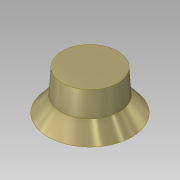
# Autodesk Inventor part: Knob
Saved by Autodesk Inventor 2016 (Build 200138000, 138)
## iProperties
Created: 2018-09-08
Part Number: Knob
Material: Generic
Document SubType Name: Modeling
Designer: Pedro Mendonça
Density: 1 g/cm^3
Appearance: Gold - Metal
Author: Pedro Mendonça
Autodesk Inventor part; units mm, degrees
ref_plane "XZ Plane" through (0, 0, 0) normal (0, 1, 0) x (-1, 0, 0)
ref_plane "XY Plane" through (0, 0, 0) normal (0, 0, 1) x (1, 0, 0)
sketch "Sketch1" plane through (0, 0, 0) normal (1, 0, 0) x (0, 1, 0)
  line L0 (0, 0) -> (0, 12.45)
  line L1 (0, 12.45) -> (8.7, 12.45)
  line L2 (8.7, 12.45) -> (9.2, 4.8665)
  line L3 (0, 0) -> (13.15, 0)
  line L4 (13.15, 0) -> (9.2, 4.8665)
  line L5 (0, -2.49) -> (0, 14.94) projected
  dimension "d5" = 12.45
  dimension "d6" = 8.7
  dimension "d7" = 7.6
  dimension "d8" = 13.15
  dimension "d10" = 9.2
  constraints: 10 end point, 1 horizontal, 1 perpendicular, 1 vertical
  measures "d5" distance of L0.start L0.end
  measures "d6" distance of L0.end L1.end
  measures "d7" distance of L1.end L2.end
  measures "d8" distance of L0.start L3.end
  measures "d10" distance from line of L2.end L0
revolve "Revolution1" add sketch "Sketch1" angle 360 about axis through (0, 0, -10) along (0, 0, 1)
sketch "Sketch2" plane through (0, 0, 0) normal (1, 0, 0) x (0, 1, 0)
  line L0 (-11.15, 0) -> (-7.2104, 4.8749)
  line L1 (-7.2173, 4.8665) -> (-6.8225, 10.8535)
  line L2 (-6.8225, 10.8535) -> (-4.8225, 10.8535)
  line L3 (-4.8225, 10.8535) -> (-4.8225, 0)
  line L4 (-11.15, 0) -> (-4.8225, 0)
  line L5 (-13.15, 0) -> (13.15, 0) projected
  line L6 (-11.15, 0) -> (-7.2173, 4.8665)
  line L7 (-6.8225, 10.8535) -> (-4.8225, 10.8535)
  line L8 (-4.8225, 0) -> (-11.15, 0)
  line L9 (0, -2.49) -> (0, 14.94) projected
  point P0 (0, 0)
  dimension "d14" = 6
  dimension "d15" = 2
  constraints: 16 end point, 2 horizontal, 2 parallel, 1 collinear
  measures "d14" distance of L1.start L1.end
  measures "d15" distance of L1.end L2.end
revolve "Revolution2" cut sketch "Sketch2" angle 360 about axis through (0, 0, -10) along (0, 0, 1)
sketch "Sketch3" plane through (0, 0, 0) normal (0, 0, -1) x (-1, 0, 0)
  circle A0 centre (0, 0) radius 3.125
  dimension "d17" = 6.25
  constraints: 1 centre point, 1 coincident
  measures "d17" diameter of A0
extrude "Extrusion1" cut sketch "Sketch3" against normal blind 8
sketch "Sketch4" plane through (0, 0, 0) normal (0, 0, -1) x (-1, 0, 0)
  circle A0 centre (0, 0) radius 3.125 projected
  circle A1 centre (0, -3.125) radius 0.485
  circle A2 centre (0.9657, -2.9721) radius 0.485
  circle A3 centre (1.8368, -2.5282) radius 0.485
  circle A4 centre (2.5282, -1.8368) radius 0.485
  circle A5 centre (2.9721, -0.9657) radius 0.485
  circle A6 centre (3.125, 0) radius 0.485
  circle A7 centre (2.9721, 0.9657) radius 0.485
  circle A8 centre (2.5282, 1.8368) radius 0.485
  circle A9 centre (1.8368, 2.5282) radius 0.485
  circle A10 centre (0.9657, 2.9721) radius 0.485
  circle A11 centre (0, 3.125) radius 0.485
  circle A12 centre (-0.9657, 2.9721) radius 0.485
  circle A13 centre (-1.8368, 2.5282) radius 0.485
  circle A14 centre (-2.5282, 1.8368) radius 0.485
  circle A15 centre (-2.9721, 0.9657) radius 0.485
  circle A16 centre (-3.125, 0) radius 0.485
  circle A17 centre (-2.9721, -0.9657) radius 0.485
  circle A18 centre (-2.5282, -1.8368) radius 0.485
  circle A19 centre (-1.8368, -2.5282) radius 0.485
  circle A20 centre (-0.9657, -2.9721) radius 0.485
  dimension "d20" = 0.97
  dimension "d23" = 360
  constraints: 20 centre point, 1 vertical alignment, 42 other
  measures "d20" diameter of A1
extrude "Extrusion2" cut sketch "Sketch4" against normal blind 8 contours A0 A6 | A0 A6 | A7 A0 | A0 A7 | A5 A0 | A0 A5 | A8 A0 | A0 A8 | A4 A0 | A0 A4 | A9 A0 | A0 A9 | A3 A0 | A0 A3 | A10 A0 | A0 A10 | A2 A0 | A0 A2 | A11 A0 | A0 A11 | A1 A0 | A0 A1 | A12 A0 | A0 A12 | A20 A0 | A0 A20 | A13 A0 | A0 A13 | A19 A0 | A0 A19 | A14 A0 | A0 A14 | A18 A0 | A0 A18 | A15 A0 | A0 A15 | A17 A0 | A0 A17 | A16 A0 | A0 A16
ref_plane "Work Plane1" through (15, 0, 0) normal (1, 0, 0) x (0, 1, 0)
sketch "Sketch5" plane through (15, 0, 0) normal (1, 0, 0) x (0, 1, 0)
  line L0 (-13.15, 0) -> (-12.9, 0)
  line L1 (-12.9, 0) -> (-12.9, 1)
  line L2 (-12.9, 1) -> (-13.15, 1)
  line L3 (-13.15, 1) -> (-13.15, 0)
  line L4 (-10.9, 0) -> (-10.65, 0)
  line L5 (-10.65, 0) -> (-10.65, 2)
  line L6 (-10.65, 2) -> (-10.9, 2)
  line L7 (-10.9, 2) -> (-10.9, 0)
  line L8 (-8.65, 0) -> (-8.4, 0)
  line L9 (-8.4, 0) -> (-8.4, 1)
  line L10 (-8.4, 1) -> (-8.65, 1)
  line L11 (-8.65, 1) -> (-8.65, 0)
  line L12 (-6.4, 0) -> (-6.15, 0)
  line L13 (-6.15, 0) -> (-6.15, 2)
  line L14 (-6.15, 2) -> (-6.4, 2)
  line L15 (-6.4, 2) -> (-6.4, 0)
  line L16 (-4.15, 0) -> (-3.9, 0)
  line L17 (-3.9, 0) -> (-3.9, 1)
  line L18 (-3.9, 1) -> (-4.15, 1)
  line L19 (-4.15, 1) -> (-4.15, 0)
  line L20 (-1.9, 0) -> (-1.65, 0)
  line L21 (-1.65, 0) -> (-1.65, 2)
  line L22 (-1.65, 2) -> (-1.9, 2)
  line L23 (-1.9, 2) -> (-1.9, 0)
  line L24 (0.35, 0) -> (0.6, 0)
  line L25 (0.6, 0) -> (0.6, 1)
  line L26 (0.6, 1) -> (0.35, 1)
  line L27 (0.35, 1) -> (0.35, 0)
  line L28 (2.6, 0) -> (2.85, 0)
  line L29 (2.85, 0) -> (2.85, 2)
  line L30 (2.85, 2) -> (2.6, 2)
  line L31 (2.6, 2) -> (2.6, 0)
  line L32 (4.85, 0) -> (5.1, 0)
  line L33 (5.1, 0) -> (5.1, 1)
  line L34 (5.1, 1) -> (4.85, 1)
  line L35 (4.85, 1) -> (4.85, 0)
  line L36 (7.1, 0) -> (7.35, 0)
  line L37 (7.35, 0) -> (7.35, 2)
  line L38 (7.35, 2) -> (7.1, 2)
  line L39 (7.1, 2) -> (7.1, 0)
  line L40 (9.35, 0) -> (9.6, 0)
  line L41 (9.6, 0) -> (9.6, 1)
  line L42 (9.6, 1) -> (9.35, 1)
  line L43 (9.35, 1) -> (9.35, 0)
  line L44 (11.6, 0) -> (11.85, 0)
  line L45 (11.85, 0) -> (11.85, 2)
  line L46 (11.85, 2) -> (11.6, 2)
  line L47 (11.6, 2) -> (11.6, 0)
  line L48 (13.85, 0) -> (14.1, 0)
  line L49 (14.1, 0) -> (14.1, 1)
  line L50 (14.1, 1) -> (13.85, 1)
  line L51 (13.85, 1) -> (13.85, 0)
  line L52 (16.1, 0) -> (16.35, 0)
  line L53 (16.35, 0) -> (16.35, 2)
  line L54 (16.35, 2) -> (16.1, 2)
  line L55 (16.1, 2) -> (16.1, 0)
  line L56 (18.35, 0) -> (18.6, 0)
  line L57 (18.6, 0) -> (18.6, 1)
  line L58 (18.6, 1) -> (18.35, 1)
  line L59 (18.35, 1) -> (18.35, 0)
  line L60 (20.6, 0) -> (20.85, 0)
  line L61 (20.85, 0) -> (20.85, 2)
  line L62 (20.85, 2) -> (20.6, 2)
  line L63 (20.6, 2) -> (20.6, 0)
  line L64 (22.85, 0) -> (23.1, 0)
  line L65 (23.1, 0) -> (23.1, 1)
  line L66 (23.1, 1) -> (22.85, 1)
  line L67 (22.85, 1) -> (22.85, 0)
  line L68 (25.1, 0) -> (25.35, 0)
  line L69 (25.35, 0) -> (25.35, 2)
  line L70 (25.35, 2) -> (25.1, 2)
  line L71 (25.1, 2) -> (25.1, 0)
  line L72 (27.35, 0) -> (27.6, 0)
  line L73 (27.6, 0) -> (27.6, 1)
  line L74 (27.6, 1) -> (27.35, 1)
  line L75 (27.35, 1) -> (27.35, 0)
  line L76 (29.6, 0) -> (29.85, 0)
  line L77 (29.85, 0) -> (29.85, 2)
  line L78 (29.85, 2) -> (29.6, 2)
  line L79 (29.6, 2) -> (29.6, 0)
  line L80 (31.85, 0) -> (32.1, 0)
  line L81 (32.1, 0) -> (32.1, 1)
  line L82 (32.1, 1) -> (31.85, 1)
  line L83 (31.85, 1) -> (31.85, 0)
  line L84 (-14.064, 4.2499) -> (-11.4376, 4.2499) construction
  line L85 (-11.4376, 4.2499) -> (-11.4376, 0.6052) construction
  line L86 (-11.4376, 0.6052) -> (-14.064, 0.6052) construction
  line L87 (-14.064, 0.6052) -> (-14.064, 4.2499) construction
  line L88 (-9.4748, 4.2276) -> (-6.8484, 4.2276) construction
  line L89 (-6.8484, 4.2276) -> (-6.8484, 0.5829) construction
  line L90 (-6.8484, 0.5829) -> (-9.4748, 0.5829) construction
  line L91 (-9.4748, 0.5829) -> (-9.4748, 4.2276) construction
  line L92 (-4.9748, 0.5829) -> (-4.9748, 4.2276) construction
  line L93 (-4.9748, 4.2276) -> (-2.3484, 4.2276) construction
  line L94 (-2.3484, 4.2276) -> (-2.3484, 0.5829) construction
  line L95 (-2.3484, 0.5829) -> (-4.9748, 0.5829) construction
  line L96 (-0.4748, 0.5829) -> (-0.4748, 4.2276) construction
  line L97 (-0.4748, 4.2276) -> (2.1516, 4.2276) construction
  line L98 (2.1516, 4.2276) -> (2.1516, 0.5829) construction
  line L99 (2.1516, 0.5829) -> (-0.4748, 0.5829) construction
  line L100 (4.0252, 0.5829) -> (4.0252, 4.2276) construction
  line L101 (4.0252, 4.2276) -> (6.6516, 4.2276) construction
  line L102 (6.6516, 4.2276) -> (6.6516, 0.5829) construction
  line L103 (6.6516, 0.5829) -> (4.0252, 0.5829) construction
  line L104 (8.5252, 0.5829) -> (8.5252, 4.2276) construction
  line L105 (8.5252, 4.2276) -> (11.1516, 4.2276) construction
  line L106 (11.1516, 4.2276) -> (11.1516, 0.5829) construction
  line L107 (11.1516, 0.5829) -> (8.5252, 0.5829) construction
  line L108 (13.0252, 0.5829) -> (13.0252, 4.2276) construction
  line L109 (13.0252, 4.2276) -> (15.6516, 4.2276) construction
  line L110 (15.6516, 4.2276) -> (15.6516, 0.5829) construction
  line L111 (15.6516, 0.5829) -> (13.0252, 0.5829) construction
  line L112 (17.5252, 0.5829) -> (17.5252, 4.2276) construction
  line L113 (17.5252, 4.2276) -> (20.1516, 4.2276) construction
  line L114 (20.1516, 4.2276) -> (20.1516, 0.5829) construction
  line L115 (20.1516, 0.5829) -> (17.5252, 0.5829) construction
  line L116 (22.0252, 0.5829) -> (22.0252, 4.2276) construction
  line L117 (22.0252, 4.2276) -> (24.6516, 4.2276) construction
  line L118 (24.6516, 4.2276) -> (24.6516, 0.5829) construction
  line L119 (24.6516, 0.5829) -> (22.0252, 0.5829) construction
  line L120 (26.5252, 0.5829) -> (26.5252, 4.2276) construction
  line L121 (26.5252, 4.2276) -> (29.1516, 4.2276) construction
  line L122 (29.1516, 4.2276) -> (29.1516, 0.5829) construction
  line L123 (29.1516, 0.5829) -> (26.5252, 0.5829) construction
  line L124 (30.2224, 0.4714) -> (30.2224, 4.1161) construction
  line L125 (30.2224, 4.1161) -> (32.8488, 4.1161) construction
  line L126 (32.8488, 4.1161) -> (32.8488, 0.4714) construction
  line L127 (32.8488, 0.4714) -> (30.2224, 0.4714) construction
  point P0 (0, 0)
  dimension "d70" = 2
  dimension "d71" = 2
  dimension "d72" = 2
  dimension "d73" = 2
  dimension "d74" = 2
  dimension "d75" = 2
  dimension "d76" = 2
  dimension "d77" = 2
  dimension "d78" = 2
  dimension "d79" = 2
  dimension "d80" = 2
  dimension "d81" = 2
  dimension "d82" = 2
  dimension "d83" = 2
  dimension "d84" = 2
  dimension "d85" = 2
  dimension "d86" = 2
  dimension "d87" = 2
  dimension "d88" = 2
  dimension "d89" = 2
  constraints: 168 end point, 42 parallel, 21 horizontal, 21 perpendicular, 22 other
  measures "d70" distance between parallel lines of L7 L1
  measures "d71" distance between parallel lines of L11 L5
  measures "d72" distance between parallel lines of L15 L9
  measures "d73" distance between parallel lines of L19 L13
  measures "d74" distance between parallel lines of L23 L17
  measures "d75" distance between parallel lines of L27 L21
  measures "d76" distance between parallel lines of L31 L25
  measures "d77" distance between parallel lines of L35 L29
  measures "d78" distance between parallel lines of L39 L33
  measures "d79" distance between parallel lines of L43 L37
  measures "d80" distance between parallel lines of L47 L41
  measures "d81" distance between parallel lines of L51 L45
  measures "d82" distance between parallel lines of L55 L49
  measures "d83" distance between parallel lines of L59 L53
  measures "d84" distance between parallel lines of L63 L57
  measures "d85" distance between parallel lines of L67 L61
  measures "d86" distance between parallel lines of L71 L65
  measures "d87" distance between parallel lines of L75 L69
  measures "d88" distance between parallel lines of L79 L73
  measures "d89" distance between parallel lines of L83 L77
body "Solid1"
